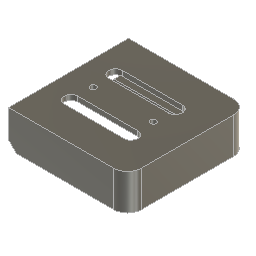
Крепление аккамулятора Bosch (Autodesk Fusion 360 design; units mm, degrees)
Autodesk Fusion 360 part; units mm, degrees
sketch "Sketch1" plane through (0, 0, 0) normal (0, 0, 1) x (1, 0, 0)
  line L0 (30, 25.7) -> (-30, 25.7)
  line L1 (-30, 25.7) -> (-30, -25.7)
  line L2 (-30, -25.7) -> (30, -25.7)
  line L3 (30, -25.7) -> (30, 25.7)
  line L4 (30, -30) -> (-30, -30)
  line L5 (-30, -35) -> (-30, 35)
  line L6 (-30, 30) -> (30, 30)
  line L7 (30, 30) -> (30, -30)
  line L8 (-30, 35) -> (27, 35)
  line L9 (35, 27) -> (35, -27)
  line L10 (-30, -35) -> (27, -35)
  arc A0 (35, 27) -> (27, 35) centre (27, 27) ccw
  arc A1 (27, -35) -> (35, -27) centre (27, -27) ccw
  circle A2 centre (-20, 0) radius 1.75
  circle A3 centre (15, 0) radius 1.75
  line L11 (-20, 9) -> (15, 9)
  arc A4 (15, 9) -> (15, 17) centre (15, 13) ccw
  line L12 (15, 17) -> (-20, 17)
  arc A5 (-20, 17) -> (-20, 9) centre (-20, 13) ccw
  line L13 (-20, 13) -> (15, 13) construction
  line L14 (1.75, 0) -> (22.5, 0)
  line L15 (-20, -9) -> (15, -9)
  arc A6 (-20, -9) -> (-20, -17) centre (-20, -13) ccw
  line L16 (15, -17) -> (-20, -17)
  arc A7 (15, -17) -> (15, -9) centre (15, -13) ccw
  dimension "d1" = 60
  dimension "d2" = 51.4
  dimension "d3" = 60
  dimension "d6" = 8
  dimension "d15" = 3.5
  dimension "d16" = 3.5
  constraint horizontal L0
  constraint perpendicular L0 L1
  constraint parallel L0 L2
  constraint parallel L1 L3
  constraint horizontal L4
  constraint perpendicular L4 L5
  constraint parallel L4 L6
  constraint parallel L5 L7
  constraint coincident L6.start L5
  constraint coincident L4.end L5
  constraint tangent L9 A0
  constraint tangent L8 A0
  constraint tangent L10 A1
  constraint tangent L9 A1
  constraint equal A0 A1
  constraint tangent L11 A4
  constraint tangent A4 L12
  constraint parallel L11 L12
  constraint tangent L12 A5
  constraint tangent L11 A5
  constraint horizontal L13
  constraint symmetric L11.start L14 L15.start
  constraint symmetric L11.end L14 L15.end
  constraint symmetric A4.end L14 L16.start
  constraint symmetric L12.end L14 A6.end
  constraint symmetric A4 L14 A7
  constraint symmetric A5 L14 A6
  measures "d1" distance of L1.end L2.end
  measures "d2" distance of L0.end L1.end
  measures "d3" distance of L4.end L6.start
  measures "d6" radius of A0
  measures "d15" diameter of A2
  measures "d16" diameter of A3
extrude "Extrude1" add sketch "Sketch1" along normal blind 5.5 contours L3 L4 L5 L6 L7 L8 L9 L10 A0 A1 | L0 L5 L6 L7 | L2 L4 L5 L7
extrude "Extrude2" add sketch "Sketch1" along normal blind 18 contours L3 L4 L5 L6 L7 L8 L9 L10 A0 A1
extrude "Extrude3" add sketch "Sketch1" along normal blind 21 and the other way blind -18
sketch "Sketch2" plane through (0, -35, 0) normal (0, -1, 0) x (1, 0, 0)
  line L0 (-30, 0) -> (27, 0)
  line L1 (27, 0) -> (27, 21)
  line L2 (27, 21) -> (-30, 21)
  line L3 (-30, 21) -> (-30, 0)
  line L4 (-30, 0) -> (-34.45, 0)
  line L5 (-34.45, 0) -> (-34.45, 4.55)
  line L6 (-30, 0) -> (-30.316, 0.3196)
  line L7 (-30.316, 0.3196) -> (-34.45, 4.55)
  line L8 (-34.45, 4.55) -> (-34.45, 21)
  line L9 (-34.45, 21) -> (-30, 21)
  line L10 (-30, 0) -> (-30, 5.5)
  line L11 (-30, 5.5) -> (-34.45, 5.5)
  dimension "d17" = 4.45
  dimension "d18" = 4.55
  dimension "d25" = 5.5
  constraint coincident L0.start L3.end
  constraint perpendicular L3 L4
  constraint perpendicular L4 L5
  constraint parallel L5 L8
  constraint coincident L2.end L3.start
  constraint perpendicular L3 L9
  constraint perpendicular L4 L10
  constraint coincident L8 L11.end
  constraint perpendicular L8 L11
  measures "d17" distance of L0.start L4.end
  measures "d18" distance of L4.end L5.end
  measures "d25" distance of L0.start L10.end
extrude "Extrude4" add sketch "Sketch2" against normal blind 5 contours L3 L6 L7 L8 L10 L11 | L3 L8 L9 L11
extrude "Extrude5" add sketch "Sketch2" along normal blind -70 and the other way blind 65 contours L3 L6 L7 L8 L10 L11 | L3 L8 L9 L11
extrude "Extrude6" add sketch "Sketch2" against normal blind 9.3 contours L3 L6 L7 L8 L10 L11
extrude "Extrude7" add sketch "Sketch2" along normal blind -65 and the other way blind 60.7 contours L3 L6 L7 L8 L10 L11
extrude "Extrude8" add 1 faces at (-30, -10, 19) along direction (-1, 0, 0) blind 4.45
chamfer "Chamfer1" distance 0.9 angle 45 2 edges at (-34.45, 27.85, 5.5) (-34.45, -27.85, 5.5)
